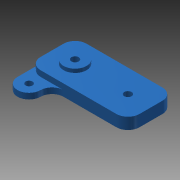
# Autodesk Inventor part: wheel tensioner
Saved by Autodesk Inventor 2013 (Build 170138000, 138)
## iProperties
Created: 2017-01-26
Part Number: wheel tensioner
Material: Generic
Document SubType Name: Modeling
Designer: Herman de Vries
Density: 1 g/cm^3
Author: Herman de Vries
Autodesk Inventor part; units mm, degrees
ref_plane "YZ Plane" through (0, 0, 0) normal (1, 0, 0) x (0, 1, 0)
ref_plane "XZ Plane" through (0, 0, 0) normal (0, 1, 0) x (-1, 0, 0)
ref_plane "XY Plane" through (0, 0, 0) normal (0, 0, 1) x (1, 0, 0)
sketch "Sketch1" plane through (0, 0, 0) normal (0, 0, 1) x (1, 0, 0)
  line L0 (0, 0) -> (43, 0)
  line L1 (43, 0) -> (43, 20)
  line L2 (43, 20) -> (0, 20)
  line L3 (0, 20) -> (0, 0)
  circle A0 centre (10, 10) radius 1.6
  circle A1 centre (33, 10) radius 1.6
  line L4 (0, -10) -> (10, -10)
  line L5 (10, -10) -> (10, 0)
  line L6 (10, 0) -> (0, 0)
  line L7 (0, 0) -> (0, -10)
  circle A2 centre (5, -5) radius 1.5
  point P0 (0, 10)
  point P1 (0, -5)
  point P2 (5, 0)
  dimension "d2" = 20
  dimension "d3" = 3.2
  dimension "d4" = 3.2
  dimension "d5" = 10
  dimension "d6" = 10
  dimension "d10" = 23
  dimension "d15" = 10
  dimension "d16" = 10
  dimension "d17" = 3
  constraints: 16 end point, 4 parallel, 3 centre point, 3 horizontal alignment, 3 midpoint, 2 horizontal, 2 perpendicular, 1 coincident, 1 vertical alignment
  measures "d2" distance of L0.end L1.end
  measures "d3" diameter of A0
  measures "d4" diameter of A1
  measures "d5" distance from line of A0.centre L3
  measures "d6" distance from line of L1 A1.centre
  measures "d10" distance of A1.centre A0.centre
  measures "d15" distance of L0.start L5.end
  measures "d16" distance of L5.end L4.end
  measures "d17" diameter of A2
extrude "Extrusion1" add sketch "Sketch1" along normal blind 5
sketch "Sketch2" plane through (0, 0, 5) normal (0, 0, 1) x (1, 0, 0)
  circle A0 centre (10, 10) radius 1.6 projected
  circle A1 centre (10, 10) radius 5
  point P0 (0, 0)
  dimension "d11" = 10
  constraints: 1 centre point, 1 coincident
  measures "d11" diameter of A1
extrude "Extrusion2" add sketch "Sketch2" along normal blind 1.6
fillet "Fillet2" radius 5 6 edges at (43, 20, 2.5) (43, 0, 2.5) (10, -10, 2.5) (0, -10, 2.5) (10, 0, 2.5) (0, 20, 2.5)
sketch "Sketch3" plane through (0, 0, 5) normal (0, 0, 1) x (1, 0, 0)
  line L0 (0, 0) -> (16.7828, 0)
  line L1 (16.7828, 0) -> (16.7828, -11.2372)
  line L2 (16.7828, -11.2372) -> (0, -11.2372)
  line L3 (0, -11.2372) -> (0, 0)
  constraints: 8 end point, 2 parallel, 1 horizontal, 1 perpendicular
extrude "Extrusion3" cut sketch "Sketch3" against normal blind 2.5
fillet "Fillet3" radius 5 1 edges at (0, 0, 3.75)
body "Solid1"
